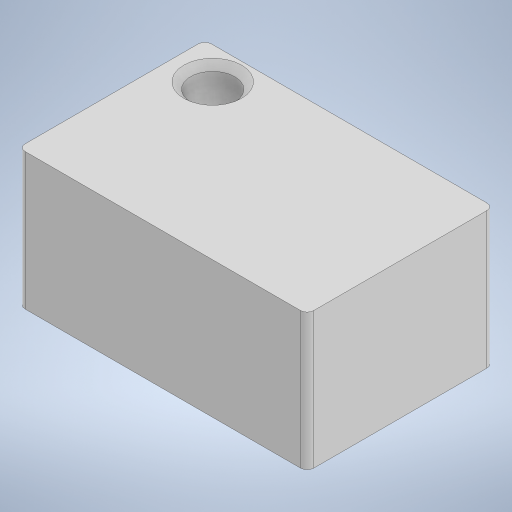
# Autodesk Inventor part: podpora_imu
Saved by Autodesk Inventor 2023.4 (Build 274418000, 418)
## iProperties
Created: 2024-10-12
Part Number: podpora_imu
Material: Generic
Document SubType Name: Modeling
Designer: komputer
Density: 1 g/cm^3
Appearance: Default
Author: komputer
Autodesk Inventor part; units mm, degrees
ref_plane "YZ Plane" through (0, 0, 0) normal (1, 0, 0) x (0, 1, 0)
ref_plane "XZ Plane" through (0, 0, 0) normal (0, 1, 0) x (-1, 0, 0)
ref_plane "XY Plane" through (0, 0, 0) normal (0, 0, 1) x (1, 0, 0)
sketch "Sketch1" plane through (0, 0, 0) normal (0, 1, 0) x (-1, 0, 0)
  line L0 (5.5664, 6.3616) -> (-16.4336, 6.3616)
  line L1 (-16.4336, 6.3616) -> (-16.4336, -7.8384)
  line L2 (-16.4336, -7.8384) -> (5.5664, -7.8384)
  line L3 (5.5664, -7.8384) -> (5.5664, 6.3616)
  point P0 (0, 0)
  dimension "d2" = 14.2
  dimension "d3" = 22
  constraints: 8 end point, 2 parallel, 1 horizontal, 1 perpendicular
  measures "d2" distance of L2.end L0.start
  measures "d3" distance of L0.start L0.end
extrude "Extrusion1" add sketch "Sketch1" along normal blind 10.4
sketch "Sketch2" plane through (0, 10.4, 0) normal (0, 1, 0) x (1, 0, 0)
  line L0 (-5.5664, -6.3616) -> (16.4336, -6.3616) projected
  line L1 (16.4336, -6.3616) -> (16.4336, 7.8384) projected
  line L2 (16.4336, 7.8384) -> (-5.5664, 7.8384) projected
  line L3 (-5.5664, 7.8384) -> (-5.5664, -6.3616) projected
  line L4 (-5.5664, -6.3616) -> (16.4336, -6.3616) projected
  line L5 (-4.3664, -6.3616) -> (-4.3664, 7.8384)
  line L6 (-5.5664, 7.8384) -> (-5.5664, -6.3616) projected
  line L7 (-5.5664, 7.2384) -> (16.4336, 7.2384)
  line L8 (16.4336, -6.3616) -> (16.4336, 7.8384) projected
  circle A0 centre (-2.5164, 5.3884) radius 1.85
  circle A1 centre (-2.5164, 5.3884) radius 1.7
  point P0 (0, 0)
  point P1 (5.4336, 7.2384)
  dimension "d4" = 1.2
  dimension "d5" = 0.6
  dimension "d6" = 3.7
  dimension "d8" = 3.4
  constraints: 4 end point, 4 point on line, 2 centre point, 2 coincident, 2 perpendicular, 2 tangent, 1 midpoint
  measures "d4" distance between parallel lines of L3 L5
  measures "d5" distance from line of L2 point (5.434, 7.238)
  measures "d6" diameter of A0
  measures "d8" diameter of A1
extrude "Extrusion2" cut sketch "Sketch2" against normal through all draft -2 contours A1
fillet "Fillet1" radius 0.5 4 edges at (16.4336, 5.2, 6.3616) (16.4336, 5.2, -7.8384) (-5.5664, 5.2, -7.8384) (-5.5664, 5.2, 6.3616)
chamfer "Chamfer1" distance 0.5 angle 45 1 edges at (-4.2164, 10.4, -5.3884)
body "Solid1"
